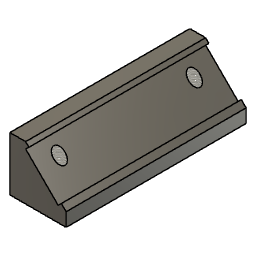
move_base_led_holder (Autodesk Fusion 360 design; units mm, degrees)
Autodesk Fusion 360 part; units mm, degrees
sketch "スケッチ1" plane through (0, 0, 0) normal (0, 0, 1) x (1, 0, 0)
  line L0 (-6, 0) -> (6.5, 0)
  line L1 (-2.5, 12) -> (-6, 12)
  line L2 (-6, 12) -> (-6, 0)
  line L3 (6.5, 0) -> (6.5, 3)
  line L4 (6.5, 3) -> (5.4393, 4.0607)
  line L5 (5.4393, 4.0607) -> (4.7322, 3.3536)
  line L6 (4.7322, 3.3536) -> (-2.4803, 10.566)
  line L7 (-2.4803, 10.566) -> (-1.7731, 11.2731)
  line L8 (-1.7731, 11.2731) -> (-2.5, 12)
  dimension "d3" = 6.5
  dimension "d4" = 6
  dimension "d13" = 12
  dimension "d19" = 1
  dimension "d20" = 10.2
  dimension "d21" = 3
  dimension "d22" = 1.5
  dimension "d23" = 1
  dimension "d24" = 45
  constraint horizontal L0
  constraint parallel L0 L1
  constraint vertical L2
  constraint coincident origin L0
  constraint perpendicular L0 L3
  constraint perpendicular L4 L5
  constraint perpendicular L5 L6
  constraint perpendicular L6 L7
  constraint perpendicular L7 L8
  constraint coincident L1.start L8.end
  measures "d3" distance of origin L0.end
  measures "d4" distance of origin L2
  measures "d13" distance of L0 L1
  measures "d19" distance of L4.end L5.end
  measures "d20" distance of L5.end L6.end
  measures "d21" distance of L0.end L3.end
  measures "d22" distance of L3.end L4.end
  measures "d23" distance of L6.end L7.end
  measures "d24" angle of L3 L4
extrude "押し出し1" add sketch "スケッチ1" along normal mid plane 40
sketch "スケッチ2" plane through (0, 0, 0) normal (0, -1, 0) x (1, 0, 0)
  line L0 (6.5, 20) -> (-6, 20)
  line L1 (-6, 20) -> (-6, -20)
  line L2 (-6, -20) -> (6.5, -20)
  line L3 (0, 15) -> (0, -15)
  line L4 (6.5, -20) -> (6.5, 20)
  dimension "d7" = 30
  constraint vertical L3
  constraint midpoint origin L3
  measures "d7" distance of L3.start L3.end
hole "穴1" at (0, 0, -15) at (0, 0, 15) direction (0, 1, 0) diameter 3 end through all
thread "ねじ1" "ISO Metric profile 3.0 M3x0.5 6H" major diameter 3.086 minor diameter 2.529 pitch 0.5 angle 60 resizes the face on face at (0.6681, 4.9414, 13.657) on face at (0.6681, 4.9414, -16.343)
